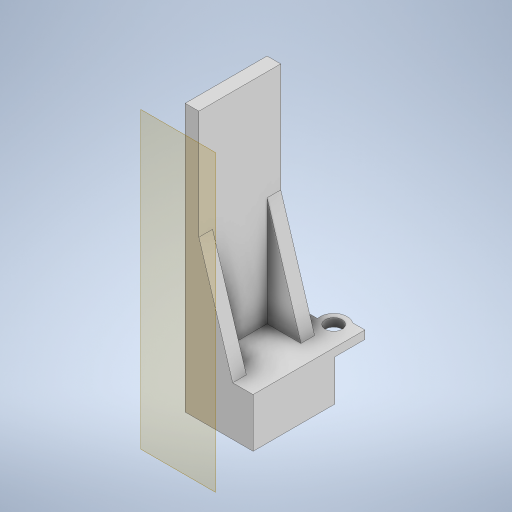
# Autodesk Inventor part: motor_limit_1
Saved by Autodesk Inventor 2024.3 (Build 283343000, 343)
## iProperties
Created: 2025-10-23
Part Number: motor_limit_1
Material: 일반
Document SubType Name: Modeling
Designer: joung
Density: 1 g/cm^3
Appearance: 기본값
Author: joung
Autodesk Inventor part; units mm, degrees
ref_plane "YZ Plane" through (0, 0, 0) normal (1, 0, 0) x (0, 1, 0)
ref_plane "XZ Plane" through (0, 0, 0) normal (0, 1, 0) x (-1, 0, 0)
ref_plane "XY Plane" through (0, 0, 0) normal (0, 0, 1) x (1, 0, 0)
sketch "스케치2" plane through (0, 0, 0) normal (0, 1, 0) x (-1, 0, 0)
  circle A0 centre (0, 0) radius 3.1
  line L0 (0, 0) -> (0, 7)
  line L1 (0, 7) -> (7.475, 7)
  line L2 (7.475, 7) -> (7.475, 1.05)
  circle A1 centre (0, 0) radius 5
  line L3 (7.475, 1.05) -> (4.8885, 1.05)
  line L4 (0, 7) -> (-7.475, 7)
  line L5 (-7.475, 7) -> (-7.475, -5)
  line L6 (-7.475, -5) -> (0, -5)
  line L7 (-7.475, -5) -> (-7.475, -4)
  line L8 (-7.475, -4) -> (-3, -4)
  dimension "d0" = 6.2
  dimension "d1" = 7
  dimension "d2" = 7.475
  dimension "d3" = 5.95
  dimension "d4" = 10
  dimension "d5" = 7.475
  dimension "d21" = 1
  constraints: 18 end point, 3 horizontal, 3 point on circle, 2 centre point, 2 coincident, 2 perpendicular, 2 vertical, 1 point on line, 1 tangent
  measures "d0" diameter of A0
  measures "d1" distance of L0.start L0.end
  measures "d2" distance of L0.end L1.end
  measures "d3" distance of L1.end L2.end
  measures "d4" diameter of A1
  measures "d5" distance of L0.end L4.end
  measures "d21" distance of L5.end L7.end
extrude "돌출1" add sketch "스케치2" along normal blind 3 contours A1 | A1 L8 L5 L4 L0 | L0 L1 L2 L3 A1
sketch "스케치3" plane through (0, 3, 0) normal (0, 1, 0) x (1, 0, 0)
  line L0 (-7.475, -7) -> (7.475, -7) projected
  line L1 (-7.475, -7) -> (7.475, -7)
  line L2 (7.475, -7) -> (7.475, -37)
  line L3 (7.475, -37) -> (-7.475, -37)
  line L4 (-7.475, -37) -> (-7.475, -7)
  point P0 (0, 0)
  dimension "d8" = 30
  constraints: 8 end point, 2 parallel, 1 horizontal, 1 perpendicular
  measures "d8" distance of L1.end L2.end
extrude "돌출2" add sketch "스케치3" against normal blind 18
sketch "스케치11" plane through (0, 3, 0) normal (0, 1, 0) x (1, 0, 0)
  line L0 (-7.475, -37) -> (7.475, -37) projected
  line L1 (0, -37) -> (-17.4, -37)
  line L2 (-17.4, -37) -> (-17.4, -1.05)
  line L3 (-17.4, -1.05) -> (0, -1.05)
  line L4 (0, -1.05) -> (0, -37)
  line L5 (-7.475, -7) -> (7.475, -7) projected
  line L6 (-17.4, -37) -> (0, -37)
  line L7 (0, -37) -> (0, -7)
  line L8 (0, -7) -> (-17.4, -7)
  line L9 (-17.4, -7) -> (-17.4, -37)
  point P0 (0, 0)
  dimension "d40" = 17.4
  constraints: 16 end point, 4 parallel, 2 horizontal, 2 midpoint, 2 perpendicular
  measures "d40" distance of L2.end L3.end
extrude "돌출9" add sketch "스케치11" along normal blind 80 and the other way blind 18 contours L1 L2 L8 L5 L4 L0
sketch "스케치12" plane through (0, 83, 0) normal (0, 1, 0) x (1, 0, 0)
  line L0 (0, -7) -> (0, -37) projected
  line L1 (-17.4, -37) -> (0, -37) projected
  line L2 (0, -7) -> (-17.4, -7)
  line L3 (-17.4, -7) -> (-17.4, -37)
  line L4 (-17.4, -37) -> (0, -37)
  line L5 (0, -37) -> (0, -7)
  line L6 (-12.4, -12) -> (-5, -12)
  line L7 (-5, -12) -> (-5, -32)
  line L8 (-5, -32) -> (-12.4, -32)
  line L9 (-12.4, -32) -> (-12.4, -12)
  line L10 (-5, -12) -> (0, -12)
  line L11 (-5, -32) -> (0, -32)
  point P0 (0, 0)
  dimension "d45" = 5
  constraints: 20 end point, 4 parallel, 4 perpendicular, 2 point on line, 1 horizontal, 3 other
  measures "d45" distance between parallel lines of L2 L6
extrude "돌출10" cut sketch "스케치12" against normal blind 80 contours L0 L11 L7 L10 | L7 L8 L9 L6
sketch "스케치13" plane through (7.475, -15, 37) normal (0, 0, 1) x (1, 0, 0)
  line L0 (-7.475, 18) -> (-7.475, 98) projected
  line L1 (-7.475, 18) -> (-19.875, 18)
  line L2 (-19.875, 18) -> (-19.875, 98)
  line L3 (-19.875, 98) -> (-19.875, 58)
  line L4 (-7.475, 18) -> (-19.875, 58)
  line L5 (-24.875, 98) -> (-7.475, 98) projected
  line L6 (-19.875, 98) -> (-7.475, 98)
  line L7 (-7.475, 98) -> (-7.475, 18)
  point P0 (-7.475, 15)
  constraints: 12 end point, 2 perpendicular, 1 collinear, 1 midpoint
extrude "돌출11" cut sketch "스케치13" against normal blind 80 contours L4 L2 L5 L0
ref_plane "작업 평면5" through (7.475, -15, 52) normal (0, 0, 1) x (1, 0, 0)
sketch "스케치4" plane through (0, 3, 0) normal (0, 1, 0) x (1, 0, 0)
  line L0 (-7.475, -1.05) -> (-7.475, -37) projected
  line L1 (7.475, -7) -> (7.475, -37) projected
  line L2 (-7.475, -37) -> (7.475, -37)
  line L3 (7.475, -37) -> (7.475, -7)
  line L4 (7.475, -7) -> (-7.475, -7)
  line L5 (-7.475, -7) -> (-7.475, -37)
  line L6 (7.475, -7) -> (4.475, -7)
  line L7 (4.475, -7) -> (4.475, -37)
  line L8 (4.475, -37) -> (7.475, -37)
  line L9 (7.475, -37) -> (7.475, -7)
  point P0 (0, 0)
  dimension "d11" = 3
  constraints: 16 end point, 4 parallel, 2 horizontal, 2 perpendicular, 1 point on line
  measures "d11" distance of L8.end L7.end
sketch "스케치5" plane through (-7.475, -15, 37) normal (0, 0, 1) x (1, 0, 0)
  line L0 (11.95, 18) -> (11.95, 88) projected
  line L1 (0, 18) -> (0, 0) projected
  line L2 (11.95, 53) -> (0, 18)
  point P0 (7.475, 15)
  constraints: 2 end point, 1 midpoint
sketch "스케치6" plane through (0, -15, 0) normal (0, -1, 0) x (1, 0, 0)
  line L0 (7.475, -4) -> (3, -4) projected
  line L1 (7.475, 37) -> (-7.475, 37) projected
  line L2 (7.475, -4) -> (7, -4)
  line L3 (7, -4) -> (7, 37)
  line L4 (7, 37) -> (7.475, 37)
  line L5 (7.475, 37) -> (7.475, -4)
  dimension "d25" = 0.475
  constraints: 8 end point, 2 parallel, 1 horizontal, 1 perpendicular, 1 point on line
  measures "d25" distance of L3.end L4.end
sketch "스케치7" plane through (0, 3, 0) normal (0, 1, 0) x (1, 0, 0)
  circle A0 centre (0, 0) radius 3.1 projected
  line L0 (0, 0) -> (25, 0)
  line L1 (25, 0) -> (25, -7)
  line L2 (7, -7) -> (25, -7)
  line L3 (25, -7) -> (25, -37)
  line L4 (25, -37) -> (7, -37)
  line L5 (7, -37) -> (7, -7)
  dimension "d26" = 25
  constraints: 12 end point, 2 horizontal, 2 parallel, 1 perpendicular, 1 point on line, 1 vertical
  measures "d26" distance of L0.start L0.end
sketch "스케치8" plane through (0, 73, 0) normal (0, 1, 0) x (1, 0, 0)
  line L0 (25, -7) -> (25, -37) projected
  line L1 (4.475, -7) -> (4.475, -37) projected
  line L2 (25, -7) -> (4.475, -7)
  line L3 (4.475, -7) -> (4.475, -37)
  line L4 (4.475, -37) -> (25, -37)
  line L5 (25, -37) -> (25, -7)
  line L6 (4.475, -10) -> (-7.475, -10) projected
  line L7 (4.475, -10) -> (20, -10)
  line L8 (20, -10) -> (20, -34)
  line L9 (20, -34) -> (4.475, -34)
  line L10 (4.475, -34) -> (4.475, -10)
  point P0 (0, 0)
  dimension "d31" = 15.525
  constraints: 16 end point, 4 parallel, 2 horizontal, 2 perpendicular
  measures "d31" distance of L8.end L9.end
sketch "스케치9" plane through (4.475, 38, 37) normal (0, 0, 1) x (1, 0, 0)
  line L0 (0, 0) -> (0, 35) projected
  line L1 (15.525, 35) -> (15.525, -35) projected
  line L2 (0, 0) -> (15.525, 35)
  line L3 (15.525, 35) -> (0, 35)
  line L4 (0, 0) -> (0, 35)
  point P0 (-4.475, -38)
  constraints: 6 end point, 2 perpendicular
sketch "스케치10" plane through (-7.475, -15, 37) normal (0, 0, 1) x (1, 0, 0)
  line L0 (27.475, 88) -> (27.475, 18) projected
  line L1 (11.95, 53) -> (0, 18) projected
  line L2 (27.475, 88) -> (0, 18)
  line L3 (0, 18) -> (27.475, 18)
  line L4 (32.475, 88) -> (27.475, 88) projected
  line L5 (27.475, 18) -> (27.475, 88)
  line L6 (27.475, 88) -> (27.475, 53)
  line L7 (0, 18) -> (27.475, 53)
  line L8 (0, 18) -> (11.95, 53)
  line L9 (27.475, 88) -> (11.95, 53)
  point P0 (7.475, 15)
  constraints: 14 end point, 1 collinear, 1 horizontal, 1 midpoint, 1 perpendicular
ref_plane "작업 평면4" through (7.475, 3, 82) normal (0, 0, -1) x (-1, 0, 0)
